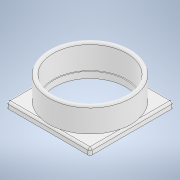
# Autodesk Inventor part: Adapter
Saved by Autodesk Inventor 2022 (Build 260153000, 153)
## iProperties
Created: 2021-10-29
Part Number: Adapter
Material: ABS Plastic
Document SubType Name: Modeling
Designer: Caleb
Density: 1.06 g/cm^3
Appearance: Smooth - White
Mass: 20.9232 g
Surface Area: 124.68 cm^2
Volume: 19.7389 cm^3
Author: Caleb
Autodesk Inventor part; units mm, degrees
ref_plane "YZ Plane" through (0, 0, 0) normal (1, 0, 0) x (0, 1, 0)
ref_plane "XZ Plane" through (0, 0, 0) normal (0, 1, 0) x (-1, 0, 0)
ref_plane "XY Plane" through (0, 0, 0) normal (0, 0, 1) x (1, 0, 0)
sketch "Sketch1" plane through (0, 0, 0) normal (0, 1, 0) x (-1, 0, 0)
  line L0 (-32.5437, -32.5438) -> (32.5438, -32.5438)
  line L1 (32.5438, -32.5438) -> (32.5438, 32.5438)
  line L2 (32.5438, 32.5438) -> (-32.5437, 32.5437)
  line L3 (-32.5437, 32.5437) -> (-32.5437, -32.5438)
  line L4 (-32.5437, -32.5438) -> (32.5438, 32.5438) construction
  line L5 (32.5438, -32.5438) -> (-32.5437, 32.5437) construction
  point P0 (0, 0)
  dimension "d0" = 65.0875
  dimension "d1" = 65.0875
  constraints: 12 end point, 2 midpoint, 2 parallel, 1 horizontal, 1 perpendicular
  measures "d0" distance of L2.end L1.end
  measures "d1" distance of L0.end L1.end
extrude "Extrusion1" add sketch "Sketch1" along normal blind 4.7625
sketch "Sketch2" plane through (0, 4.7625, 0) normal (0, 1, 0) x (1, 0, 0)
  circle A0 centre (0, 0) radius 28.575
  circle A1 centre (0, 0) radius 31.75
  dimension "d4" = 57.15
  dimension "d5" = 3.175
  constraints: 2 centre point, 2 coincident
  measures "d4" diameter of A0
  measures "d5" radial gap between concentric circles of A1 A0
extrude "Extrusion2" add sketch "Sketch2" along normal blind 19.05
sketch "Sketch3" plane through (0, 4.7625, 0) normal (0, 1, 0) x (1, 0, 0)
  circle A0 centre (0, 0) radius 27.7812
  dimension "d12" = 55.5625
  constraints: 1 centre point, 1 coincident
  measures "d12" diameter of A0
extrude "Extrusion3" cut sketch "Sketch3" against normal through all
fillet "Fillet1" radius 1.5875 1 edges at (32.5437, 4.7625, 0)
fillet "Fillet2" radius 1.5875 11 edges at (32.0788, 4.2975, 32.5437) (32.5437, 1.5875, 32.5437) (-0.7938, 4.7625, 32.5437) (-32.5438, 4.7625, 0) (-32.5438, 2.3813, 32.5438) (-32.5438, 2.3813, -32.5438) (32.0788, 4.2975, -32.5438) (32.5437, 1.5875, -32.5438) (-0.7938, 4.7625, -32.5438) (-31.75, 23.8125, 0) (-28.575, 23.8125, 0)
body "Solid1"
